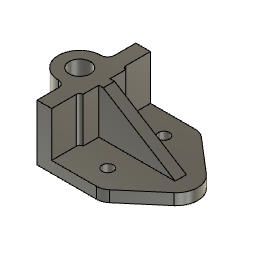
A3 (Autodesk Fusion 360 design; units mm, degrees)
Autodesk Fusion 360 part; units mm, degrees
sketch "Sketch1" plane through (0, 0, 0) normal (0, 0, 1) x (1, 0, 0)
  line L0 (12.9814, 44) -> (-40, 44)
  line L1 (-40, -44) -> (12.9814, -44)
  circle A0 centre (4, -25) radius 5
  circle A1 centre (4, 25) radius 5
  line L2 (40, -25) -> (52.3485, -14.44)
  line L3 (40, 25) -> (52.3485, 14.44)
  line L4 (40, 25) -> (21.4304, 40.88)
  line L5 (40, -25) -> (21.4304, -40.88)
  circle A2 centre (-46, 0) radius 9.5
  arc A3 (-40, -25) -> (-46, -19) centre (-46, -25) ccw
  arc A4 (52.3485, -14.44) -> (52.3485, 14.44) centre (40, 0) ccw
  arc A5 (12.9814, -44) -> (21.4304, -40.88) centre (12.9814, -31) ccw
  line L6 (-40, -25) -> (-40, -44)
  arc A6 (-46, 19) -> (-46, -19) centre (-46, 0) ccw
  line L7 (-40, 44) -> (-40, 25)
  line L8 (-40, 19) -> (-40, 18.0278)
  arc A7 (-46, 19) -> (-40, 25) centre (-46, 25) ccw
  arc A8 (21.4304, 40.88) -> (12.9814, 44) centre (12.9814, 31) ccw
  line L9 (-40, 0) -> (-36.5, 0) construction
  line L10 (0, 0) -> (4, 0) construction
  line L11 (4, 20) -> (4, 19) construction
  line L12 (20.8025, 19) -> (-35, 19) construction
  line L13 (-35, -19) -> (20, -19) construction
  line L14 (-20, -5) -> (-20, 5)
  line L15 (-24, 5) -> (-20, 5)
  line L16 (-24, -5) -> (-20, -5)
  line L17 (-24, 19) -> (-24, 5)
  line L18 (-24, -5) -> (-24, -19)
  arc A9 (-24, -19) -> (-27, -22) centre (-24, -22) ccw
  arc A10 (-27, 22) -> (-24, 19) centre (-24, 22) ccw
  line L19 (-27, 44) -> (-27, 22)
  line L20 (-27, -22) -> (-27, -44)
  line L21 (-40, 44) -> (-27, 44)
  line L22 (-40, -44) -> (-27, -44)
  line L23 (-70, 0) -> (52.6501, 0) construction
  dimension "d2" = 88
  dimension "d3" = 19
  dimension "d8" = 10
  dimension "d9" = 10
  dimension "d13" = 19
  dimension "d14" = 19
  dimension "d15" = 6
  dimension "d16" = 6
  dimension "d19" = 13
  dimension "d20" = 16
  dimension "d21" = 19
  dimension "d22" = 19
  dimension "d23" = 3
  dimension "d24" = 3
  dimension "d25" = 20
  dimension "d26" = 5
  dimension "d27" = 5
  dimension "d46" = 44
  dimension "d47" = 44
  constraint horizontal L0
  constraint perpendicular L0 L7
  constraint parallel L0 L1
  constraint coincident A3.start L7
  constraint tangent L2 A4
  constraint tangent L3 A4
  constraint parallel L3 L4
  constraint parallel L2 L5
  constraint concentric A2 A6
  constraint tangent L7 A7
  constraint tangent A3 L7
  constraint collinear L6 L7
  constraint collinear L7 L8
  constraint collinear L9 L10
  constraint coincident A1 L11.start
  constraint coincident L0 L19.start
  constraint coincident L1 L20.end
  constraint perpendicular L1 L19
  constraint perpendicular L1 L17
  constraint perpendicular L12 L17
  constraint perpendicular L13 L17
  constraint tangent A9 L19
  constraint tangent L13 A9
  constraint tangent A10 L19
  constraint tangent L12 A10
  constraint parallel L14 L17
  constraint perpendicular L14 L15
  constraint coincident L16.start L17
  constraint perpendicular L16 L17
  constraint coincident A2 L9.end
  constraint collinear L17 L18
  constraint coincident L13 L18.end
  constraint coincident A9.end L19
  constraint coincident L12 L17.start
  constraint collinear L19 L20
  constraint horizontal L23
  measures "d2" distance of L0.end L1.start
  measures "d3" radius of A4
  measures "d8" diameter of A0
  measures "d9" diameter of A1
  measures "d13" diameter of A2
  measures "d14" radius of A6
  measures "d15" radius of A7
  measures "d16" radius of A3
  measures "d19" distance of L7 L19
  measures "d20" distance of L7 L17
  measures "d21" distance of L9 L12
  measures "d22" distance of L9 L13
  measures "d23" radius of A9
  measures "d24" radius of A10
  measures "d25" distance of L7 L14
  measures "d26" distance of L9 L15
  measures "d27" distance of L9 L16
  measures "d46" distance of L1 L23
  measures "d47" distance of L0 L23
extrude "Extrude1" add sketch "Sketch1" along normal blind 10
sketch "Sketch2" plane through (0, 0, 10) normal (0, 0, 1) x (-1, 0, 0)
  circle A0 centre (-4, -25) radius 5
  circle A1 centre (-4, 25) radius 5
  circle A2 centre (46, 0) radius 9.5
  line L0 (-52.3485, -14.44) -> (-21.4304, -40.88)
  arc A3 (-21.4304, -40.88) -> (-12.9814, -44) centre (-12.9814, -31) ccw
  line L1 (-12.9814, -44) -> (40, -44)
  line L2 (40, -44) -> (40, -25)
  arc A4 (46, -19) -> (40, -25) centre (46, -25) ccw
  arc A5 (46, -19) -> (46, 19) centre (46, 0) ccw
  arc A6 (40, 25) -> (46, 19) centre (46, 25) ccw
  line L3 (40, 25) -> (40, 44)
  line L4 (40, 44) -> (-12.9814, 44)
  arc A7 (-12.9814, 44) -> (-21.4304, 40.88) centre (-12.9814, 31) ccw
  line L5 (-21.4304, 40.88) -> (-52.3485, 14.44)
  arc A8 (-52.3485, 14.44) -> (-52.3485, -14.44) centre (-40, 0) ccw
  line L6 (40, -44) -> (27, -44)
  line L7 (24, -19) -> (24, -5)
  line L8 (20, -5) -> (20, 5)
  line L9 (24, 5) -> (24, 19)
  circle A9 centre (46, 0) radius 9.5
  line L10 (40, 44) -> (27, 44)
  line L11 (40, 44) -> (40, 25)
  line L12 (40, -44) -> (40, -25)
  arc A10 (40, 25) -> (46, 19) centre (46, 25) ccw
  arc A11 (46, -19) -> (46, 19) centre (46, 0) ccw
  line L13 (40, -44) -> (40, -25) construction
  line L14 (40, 25) -> (40, 44) construction
  arc A12 (24, 19) -> (27, 22) centre (24, 22) ccw
  arc A13 (46, -19) -> (40, -25) centre (46, -25) ccw
  arc A14 (27, -22) -> (24, -19) centre (24, -22) ccw
  line L15 (24, 5) -> (20, 5)
  line L16 (24, -5) -> (20, -5)
  line L17 (27, -44) -> (27, -22) construction
  line L18 (27, 22) -> (27, 44) construction
  line L19 (27, -44) -> (27, -22)
  line L20 (27, 22) -> (27, 44)
  dimension "d28" = 13
  dimension "d35" = 3
  dimension "d36" = 3
  dimension "d37" = 19
  dimension "d39" = 6
  dimension "d40" = 6
  constraint coincident L1.end L2.start
  constraint coincident L3.end L4.start
  constraint coincident L1 L6.end
  constraint coincident L4 L10.end
  constraint perpendicular L4 L17
  constraint tangent A12 L19
  constraint tangent A14 L19
  constraint coincident A6.start L3.start
  constraint coincident L2.end A4.end
  constraint tangent L13 A13
  constraint tangent A10 L13
  constraint collinear L13 L14
  constraint coincident A12.end L17
  constraint perpendicular L8 L15
  constraint perpendicular L8 L16
  constraint collinear L17 L18
  constraint collinear L19 L20
  measures "d28" distance of L13 L17
  measures "d35" radius of A12
  measures "d36" radius of A14
  measures "d37" diameter of A9
  measures "d39" radius of A13
  measures "d40" radius of A10
extrude "Extrude2" add sketch "Sketch2" along normal blind 40 contours L1 L2 A4 A5 A6 L3 L4 L6 L7 L8 L9 L10 L11 L12 A10 A11 A12 A13 A14 L15 L16 L19 L20
sketch "Sketch3" plane through (0, 0, 0) normal (0, 1, 0) x (1, 0, 0)
  line L0 (-20, -50) -> (-20, -10)
  line L1 (-20, -10) -> (44, -10)
  line L2 (44, -10) -> (-20, -50)
  dimension "d43" = 64
  constraint vertical L0
  constraint perpendicular L0 L1
  measures "d43" distance of L0.end L1.end
extrude "Extrude3" add sketch "Sketch3" along normal mid plane 10
equation "d20 = 13 mm + 3 mm"
equation "d43 = 67 mm - 3 mm"
named bodies: "A3"
